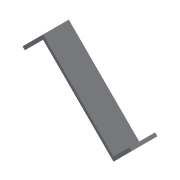
# Autodesk Inventor part: LoadSlideBracket
Saved by Autodesk Inventor 2015 (Build 190159000, 159)
## iProperties
Created: 2015-03-06
Part Number: LoadSlideBracket
Material: Generic
Document SubType Name: Modeling
Designer: Jaden
Density: 1 g/cm^3
Appearance: Default
Author: Jaden
Autodesk Inventor part; units mm, degrees
ref_plane "YZ Plane" through (0, 0, 0) normal (1, 0, 0) x (0, 1, 0)
ref_plane "XZ Plane" through (0, 0, 0) normal (0, 1, 0) x (-1, 0, 0)
ref_plane "XY Plane" through (0, 0, 0) normal (0, 0, 1) x (1, 0, 0)
sketch "Sketch1" plane through (0, 0, 0) normal (0, 0, 1) x (1, 0, 0)
  line L0 (0, 0) -> (17.9605, 17.9605)
  line L1 (0, 0) -> (25.4, 0) construction
  line L2 (17.9605, 17.9605) -> (87.3779, -51.4569)
  line L3 (87.3779, -51.4569) -> (105.3384, -33.4964)
  line L4 (105.3384, -33.4964) -> (103.0933, -31.2513)
  line L5 (103.0933, -31.2513) -> (87.3779, -46.9667)
  line L6 (87.3779, -46.9667) -> (17.9605, 22.4506)
  line L7 (17.9605, 22.4506) -> (-2.2451, 2.2451)
  line L8 (-2.2451, 2.2451) -> (0, 0)
  dimension "d14" = 25.4
  dimension "d15" = 45
  dimension "d16" = 98.171
  dimension "d17" = 25.4
  dimension "d18" = 3.175
  dimension "d19" = 22.225
  dimension "d20" = 90
  dimension "d21" = 98.171
  constraints: 18 end point, 6 perpendicular, 1 equal length, 1 horizontal
  measures "d14" distance of L0.start L0.end
  measures "d15" angle of L1 L0
  measures "d16" distance of L0.end L2.end
  measures "d17" distance of L2.end L3.end
  measures "d18" distance of L3.end L4.end
  measures "d19" distance of L4.end L5.end
  measures "d20" angle of L5 L4
  measures "d21" distance of L5.end L6.end
extrude "Extrusion1" add sketch "Sketch1" along normal blind 25.4
body "Solid1"
